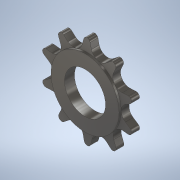
# Autodesk Inventor part: 19mmSprocket
Saved by Autodesk Inventor 2020.3 (Build 243373000, 373)
## iProperties
Created: 2019-01-20
Part Number: 19mmSprocket
Material: Steel, High Strength, Low Alloy
Document SubType Name: Modeling
Designer: Martin_
Density: 7.85 g/cm^3
Appearance: Steel - Polished
Author: Martin_
Autodesk Inventor part; units mm, degrees
ref_plane "YZ Plane" through (0, 0, 0) normal (1, 0, 0) x (0, 1, 0)
ref_plane "XZ Plane" through (0, 0, 0) normal (0, 1, 0) x (-1, 0, 0)
ref_plane "XY Plane" through (0, 0, 0) normal (0, 0, 1) x (1, 0, 0)
sketch "Náčrt1" plane through (0, 0, 0) normal (0, 0, 1) x (1, 0, 0)
  circle A0 centre (5.9788, 19.0657) radius 4.25
  line L0 (-2.2707, 17.8135) -> (1.9175, 17.8135)
  line L1 (-2.2707, 17.8135) -> (-0.7533, 23.3238)
  line L2 (-0.7533, 23.3238) -> (0.2222, 23.323)
  line L3 (1.9175, 17.8135) -> (0.7668, 23.3261)
  line L4 (0.7668, 23.3261) -> (0.2222, 23.323)
  line L5 (-12.3076, 13.0767) -> (-14.3188, 18.4266)
  line L6 (-14.3188, 18.4266) -> (-13.5292, 18.9993)
  line L7 (-13.0904, 19.3219) -> (-13.5292, 18.9993)
  line L8 (-8.9192, 15.5385) -> (-13.0904, 19.3219)
  circle A1 centre (-6.3696, 18.9388) radius 4.25
  line L9 (-17.6434, 3.3451) -> (-22.415, 6.491)
  line L10 (-22.415, 6.491) -> (-22.1129, 7.4186)
  line L11 (-21.9475, 7.9374) -> (-22.1129, 7.4186)
  line L12 (-16.3491, 7.3283) -> (-21.9475, 7.9374)
  circle A2 centre (-16.285, 11.5778) radius 4.25
  line L13 (-16.24, -7.6643) -> (-21.9494, -7.9238)
  line L14 (-21.9494, -7.9238) -> (-22.2502, -6.9959)
  line L15 (-22.4214, -6.4789) -> (-22.2502, -6.9959)
  line L16 (-17.5342, -3.681) -> (-22.4214, -6.4789)
  circle A3 centre (-19.9802, -0.2054) radius 4.25
  line L17 (-8.6335, -15.7461) -> (-13.1, -19.3121)
  line L18 (-13.1, -19.3121) -> (-13.8887, -18.7381)
  line L19 (-14.3311, -18.4205) -> (-13.8887, -18.7381)
  line L20 (-12.0218, -13.2844) -> (-14.3311, -18.4205)
  circle A4 centre (-16.0435, -11.9102) radius 4.25
  line L21 (2.2707, -17.8135) -> (0.7533, -23.3238)
  line L22 (0.7533, -23.3238) -> (-0.2222, -23.323)
  line L23 (-0.7668, -23.3261) -> (-0.2222, -23.323)
  line L24 (-1.9175, -17.8135) -> (-0.7668, -23.3261)
  circle A5 centre (-5.9788, -19.0657) radius 4.25
  line L25 (12.3076, -13.0767) -> (14.3188, -18.4266)
  line L26 (14.3188, -18.4266) -> (13.5292, -18.9993)
  line L27 (13.0904, -19.3219) -> (13.5292, -18.9993)
  line L28 (8.9192, -15.5385) -> (13.0904, -19.3219)
  circle A6 centre (6.3696, -18.9388) radius 4.25
  line L29 (17.6434, -3.3451) -> (22.415, -6.491)
  line L30 (22.415, -6.491) -> (22.1129, -7.4186)
  line L31 (21.9475, -7.9374) -> (22.1129, -7.4186)
  line L32 (16.3491, -7.3283) -> (21.9475, -7.9374)
  circle A7 centre (16.285, -11.5778) radius 4.25
  line L33 (16.24, 7.6643) -> (21.9494, 7.9238)
  line L34 (21.9494, 7.9238) -> (22.2502, 6.9959)
  line L35 (22.4214, 6.4789) -> (22.2502, 6.9959)
  line L36 (17.5342, 3.681) -> (22.4214, 6.4789)
  circle A8 centre (19.9802, 0.2054) radius 4.25
  line L37 (8.6335, 15.7461) -> (13.1, 19.3121)
  line L38 (13.1, 19.3121) -> (13.8887, 18.7381)
  line L39 (14.3311, 18.4205) -> (13.8887, 18.7381)
  line L40 (12.0218, 13.2844) -> (14.3311, 18.4205)
  circle A9 centre (16.0435, 11.9102) radius 4.25
  line L41 (8.6345, 15.7476) -> (12.0218, 13.2844)
  line L42 (12.0218, 13.2844) -> (16.2247, 7.6641)
  line L43 (16.2247, 7.6641) -> (17.5342, 3.681)
  line L44 (17.5342, 3.681) -> (17.6438, -3.3448)
  line L45 (17.6438, -3.3448) -> (17.711, -3.3897)
  line L46 (17.6438, -3.3448) -> (16.3491, -7.3283)
  line L47 (16.3491, -7.3283) -> (12.3076, -13.0753)
  line L48 (12.3076, -13.0767) -> (12.3076, -13.0753)
  line L49 (12.3076, -13.0753) -> (8.9192, -15.5385)
  line L50 (8.9192, -15.5385) -> (2.2704, -17.8165)
  line L51 (-1.9175, -17.8135) -> (-8.6347, -15.7478)
  line L52 (-8.6335, -15.7461) -> (-8.6347, -15.7478)
  line L53 (-8.6347, -15.7478) -> (-12.0218, -13.2844)
  line L54 (-12.0218, -13.2844) -> (-16.2418, -7.6649)
  line L55 (-16.24, -7.6643) -> (-16.2418, -7.6649)
  line L56 (-16.2418, -7.6649) -> (-17.5342, -3.681)
  line L57 (-17.3733, 3.1516) -> (-17.3727, 3.1507)
  line L58 (-16.3491, 7.3283) -> (-12.3089, 13.0788)
  line L59 (-12.3089, 13.0788) -> (-12.3076, 13.0767)
  line L60 (-12.3089, 13.0788) -> (-8.9192, 15.5385)
  line L61 (-8.9192, 15.5385) -> (-2.2713, 17.8133)
  line L62 (-2.2713, 17.8133) -> (-2.2707, 17.8135)
  line L63 (-17.5342, -3.681) -> (-17.6456, 3.346)
  line L64 (-17.6456, 3.346) -> (-17.6434, 3.3451)
  line L65 (-17.6434, 3.3451) -> (-16.3491, 7.3283)
  line L66 (2.2704, -17.8165) -> (2.2699, -17.8164)
  line L67 (2.2699, -17.8164) -> (-1.9175, -17.8135)
  line L68 (2.2492, -17.8916) -> (2.2704, -17.8165)
  line L69 (1.9175, 17.8135) -> (8.6345, 15.7476)
  line L70 (8.6351, 15.7474) -> (8.6345, 15.7476)
  line L71 (17.5369, 3.5092) -> (17.5342, 3.681)
  line L72 (16.2364, 7.6641) -> (16.2247, 7.6641)
  line L73 (16.2364, 7.6641) -> (16.2402, 7.6643)
  point P0 (0, 0)
  point P1 (5.9788, 14.8157)
  point P2 (-3.8715, 15.5005)
  point P3 (-12.243, 10.2645)
  point P4 (-15.9382, 1.1079)
  point P5 (-13.5454, -8.4719)
  point P6 (-5.9788, -14.8157)
  point P7 (3.8715, -15.5005)
  point P8 (12.243, -10.2645)
  point P9 (15.9382, -1.1079)
  point P10 (13.5454, 8.4719)
  dimension "d10" = 360
  dimension "d82" = 8.5
  constraints: 148 end point, 32 point on circle, 10 centre point, 8 point on line, 3 collinear, 2 horizontal, 1 coincident, 1 perpendicular, 1 vertical, 121 other
  measures "d82" diameter of A0
extrude "Extrusion1" add sketch "Náčrt1" along normal blind 3.6 contours L0 L1 L2 L4 L3 A0 | A0 L41 A9 L43 A8 L46 A7 L49 A6 L21 L67 A5 L53 A4 L56 A3 L65 A2 L5 L60 A1 L0 | A0 L3 | L37 L38 L39 L40 A9 L41 | A9 L40 | A1 L8 | L60 L5 L6 L7 L8 A1 | A9 L33 L34 L35 L36 A8 L43 | A8 L36 | A2 L65 L9 L10 L11 L12 | L12 A2 | L29 L30 L31 L32 A7 L46 | A7 L32 | L25 L26 L27 L28 A6 L49 | A3 L56 L13 L14 L15 L16 | L16 A3 | A6 L28 | L21 L22 L23 L24 A5 L67 | A4 L53 L17 L18 L19 L20 | L20 A4 | A5 L24
fillet "Fillet1" radius 1.5 30 edges at (-0.7533, 23.3238, 1.8) (0.2222, 23.323, 1.8) (0.7668, 23.3261, 1.8) (13.1, 19.3121, 1.8) (13.8887, 18.7381, 1.8) (14.3311, 18.4205, 1.8) (-13.0904, 19.3219, 1.8) (-13.5292, 18.9993, 1.8) (-14.3188, 18.4266, 1.8) (-21.9475, 7.9374, 1.8) (-22.1129, 7.4186, 1.8) (-22.415, 6.491, 1.8) (-22.4214, -6.4789, 1.8) (-22.2502, -6.9959, 1.8) (-21.9494, -7.9238, 1.8) (-14.3311, -18.4205, 1.8) (-13.8887, -18.7381, 1.8) (-13.1, -19.3121, 1.8) (-0.7668, -23.3261, 1.8) (-0.2222, -23.323, 1.8) (0.7533, -23.3238, 1.8) (13.0904, -19.3219, 1.8) (13.5292, -18.9993, 1.8) (14.3188, -18.4266, 1.8) (21.9475, -7.9374, 1.8) (22.1129, -7.4186, 1.8) (22.415, -6.491, 1.8) (22.4214, 6.4789, 1.8) (22.2502, 6.9959, 1.8) (21.9494, 7.9238, 1.8)
sketch "Sketch2" plane through (0, 0, 3.6) normal (0, 0, 1) x (1, 0, 0)
  circle A0 centre (0, 0) radius 15.7312
  arc A1 (16.3491, -7.3283) -> (12.3076, -13.0753) centre (16.285, -11.5778) ccw projected
  constraints: 1 centre point, 1 coincident, 1 tangent
extrude "Extrusion2" add sketch "Sketch2" along normal blind 1
sketch "Sketch3" plane through (0, 0, 4.6) normal (0, 0, 1) x (1, 0, 0)
  line L0 (-4, -5) -> (4, 5) construction
  line L1 (4, -5) -> (-4, 5) construction
  circle A0 centre (0, 0) radius 9.5
  dimension "d101" = 19
  constraints: 4 end point, 2 midpoint, 1 centre point, 1 coincident
  measures "d101" diameter of A0
extrude "Extrusion3" cut sketch "Sketch3" against normal blind 10
